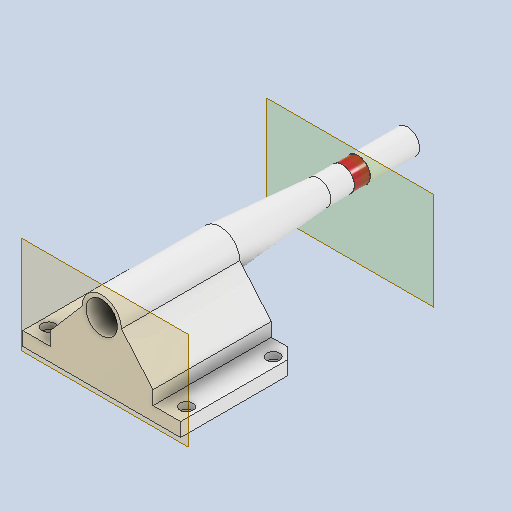
# Autodesk Inventor part: Guide
Saved by Autodesk Inventor 2024 (Build 280153000, 153)
## iProperties
Created: 2021-10-05
Part Number: Guide
Material: PBT-Kunststoff
Document SubType Name: Modeling
Designer: espen
Density: 1.31 g/cm^3
Appearance: Glatt - Weiß
Mass: 141.322 g
Surface Area: 254.19 cm^2
Volume: 107.879 cm^3
ToolGuidance_Base_Thickness: 7,000 mm
Guidacne_fixHoleDist: 70,000 mm
Author: espen
Autodesk Inventor part; units mm, degrees
ref_plane "YZ Plane" through (0, 0, 0) normal (1, 0, 0) x (0, 1, 0)
ref_plane "XZ Plane" through (0, 0, 0) normal (0, 1, 0) x (-1, 0, 0)
ref_plane "XY Plane" through (0, 0, 0) normal (0, 0, 1) x (1, 0, 0)
sketch "Sketch1" plane through (0, 0, 0) normal (0, 0, 1) x (1, 0, 0)
  arc A0 (10, 32.7) -> (-10, 32.7) centre (0, 32.7) ccw
  line L0 (-10, 32.7) -> (-26, 14)
  line L1 (-26, 14) -> (-26, 7)
  line L2 (-26, 7) -> (-40, 7)
  line L3 (-40, 7) -> (-40, 0)
  line L4 (-40, 0) -> (0, 0)
  line L5 (0, 32.7) -> (0, 0) construction
  line L6 (10, 32.7) -> (26, 14)
  line L7 (26, 14) -> (26, 7)
  line L8 (26, 7) -> (40, 7)
  line L9 (40, 7) -> (40, 0)
  line L10 (40, 0) -> (0, 0)
  line L11 (-10, 32.7) -> (10, 32.7) construction
  dimension "d4" = 10
  dimension "d5" = 80
  dimension "ToolGuidance_Base_Thickness" = 7
  dimension "d7" = 7
  dimension "d8" = 32.7
  dimension "d9" = 14
  dimension "d11" = 0
  constraints: 24 end point, 4 symmetric about line, 3 perpendicular, 2 point on circle, 2 vertical, 1 centre point, 1 coincident, 1 horizontal, 1 midpoint, 1 point on line
  measures "d4" radius of A0
  measures "d5" diameter of L3 L5
  measures "ToolGuidance_Base_Thickness" distance between parallel lines of L8 L10
  measures "d7" distance from line of L6.end L8
  measures "d8" distance from line of L10 A0.centre
  measures "d9" distance between parallel lines of L7 L9
  measures "d11" distance from line of L4.end L5
extrude "Extrusion1" add sketch "Sketch1" against normal blind 60
sketch "Sketch2" plane through (0, 0, 0) normal (0, 0, 1) x (1, 0, 0)
  arc A0 (10, 32.7) -> (-10, 32.7) centre (0, 32.7) ccw projected
  circle A1 centre (0, 32.7) radius 8
  point P0 (0, 0)
  dimension "d16" = 16
  constraints: 1 centre point, 1 coincident
  measures "d16" diameter of A1
extrude "Extrusion2" cut sketch "Sketch2" against normal blind 20
sketch "Sketch3" plane through (0, 0, -60) normal (0, 0, -1) x (-1, 0, 0)
  circle A0 centre (0, 32.7) radius 8 projected
  circle A1 centre (0, 32.7) radius 4.25
  point P0 (0, 0)
  dimension "d19" = 8.5
  constraints: 1 centre point, 1 coincident
  measures "d19" diameter of A1
extrude "Extrusion3" cut sketch "Sketch3" against normal blind 60 contours A1
sketch "Sketch4" plane through (-40, 7, 0) normal (0, 1, 0) x (1, 0, 0)
  circle A0 centre (5, 52) radius 2.25 construction
  line L0 (0, 60) -> (14, 60) construction
  line L1 (0, 0) -> (0, 60) construction
  circle A1 centre (5, 8) radius 2.25 construction
  line L2 (96, 0) -> (-16, 0) construction
  line L3 (40, 60) -> (40, 0) construction
  circle A2 centre (75, 52) radius 2.25 construction
  circle A3 centre (75, 8) radius 2.25 construction
  line L4 (80, 0) -> (80, 60) construction
  line L5 (66, 60) -> (80, 60) construction
  line L6 (75, 52) -> (75, 8) construction
  line L7 (5, 52) -> (5, 8) construction
  line L8 (0, 0) -> (0, 60) construction
  point P0 (73, 60)
  point P1 (7, 60)
  dimension "d25" = 4.5
  dimension "d26" = 8
  dimension "d28" = 4.5
  dimension "d29" = 8
  dimension "d54" = 44
  dimension "Guidacne_fixHoleDist" = 70
  constraints: 6 end point, 4 centre point, 4 coincident, 2 midpoint, 2 symmetric about line, 1 parallel, 1 point on line, 1 vertical, 2 other
  measures "d25" diameter of A0
  measures "d26" distance from line of A0.centre L0
  measures "d28" diameter of A1
  measures "d29" distance from line of A1.centre L2
  measures "d54" distance of A0.centre A1.centre
  measures "Guidacne_fixHoleDist" distance between parallel lines of L6 L7
hole "Bohrung1" at (35, 7, -52) at (35, 7, -8) at (-35, 7, -8) at (-35, 7, -52) direction (0, -1, 0) diameter 3.4 end through all counterbore diameter 6.5 counterbore depth 3.4 clearance for "Inbusschraube DIN EN ISO 4762" size "M3" standard "DIN"
sketch "Sketch5" plane through (0, 0, 0) normal (1, 0, 0) x (0, 1, 0)
  line L0 (32.7, 0) -> (32.7, -60) projected
  line L1 (32.7, 0) -> (32.7, -180.9299)
  line L2 (32.7, -60) -> (42.7, -60) projected
  line L3 (42.7, -60) -> (38.95, -110)
  line L4 (38.95, -110) -> (38.95, -155)
  line L5 (36.95, -60) -> (36.95, -20) projected
  line L6 (36.95, -60) -> (36.95, -155)
  line L7 (36.95, -155) -> (38.95, -155)
  line L8 (42.7, 0) -> (32.7, 0) projected
  point P0 (0, 0)
  dimension "d34" = 2
  dimension "d35" = 155
  dimension "d36" = 110
  constraints: 10 end point, 2 perpendicular, 2 point on line, 1 collinear, 1 parallel
  measures "d34" distance between parallel lines of L6 L4
  measures "d35" distance from line of L4.end L8
  measures "d36" distance from line of L3.end L8
revolve "Revolution1" add sketch "Sketch5" angle 360 about axis through (0, 32.7, 0) along (0, 0, -1)
sketch "Sketch6" plane through (0, 0, 0) normal (1, 0, 0) x (0, 1, 0)
  line L0 (32.7, 0) -> (32.7, -60) projected
  line L1 (32.7, -41.8536) -> (32.7, 16.9969)
  line L2 (24.7, -20) -> (40.7, -20) projected
  line L3 (40.7, -20) -> (36.95, -33.9952)
  line L4 (36.95, -155) -> (36.95, -20) projected
  line L5 (28.45, -20) -> (36.95, -20) projected
  line L6 (36.95, -33.9952) -> (36.95, -20)
  line L7 (36.95, -20) -> (40.7, -20)
  line L8 (36.95, -33.9952) -> (36.95, -20)
  line L9 (40.7, -20) -> (36.95, -20)
  point P0 (0, 0)
  dimension "d38" = 15
  constraints: 12 end point, 2 collinear, 2 perpendicular, 2 point on line, 1 vertical
  measures "d38" angle of L4 L3
revolve "Revolution2" cut sketch "Sketch6" angle 360 about axis through (0, 32.7, -41.8536) along (0, 0, 1)
sketch "Sketch7" plane through (0, 0, 0) normal (1, 0, 0) x (0, 1, 0)
  line L0 (26.45, -110) -> (38.95, -110) projected
  line L1 (32.7, -110) -> (32.7, -160.0229)
  line L2 (38.95, -110) -> (38.95, -155) projected
  line L3 (38.95, -122) -> (38.85, -122)
  line L4 (38.85, -122) -> (38.85, -130)
  line L5 (38.85, -130) -> (38.95, -130)
  line L6 (38.95, -130) -> (38.95, -122)
  line L7 (42.7, 0) -> (32.7, 0) projected
  point P0 (0, 0)
  dimension "d40" = 0.1
  dimension "d41" = 122
  dimension "d42" = 8
  constraints: 10 end point, 2 parallel, 1 horizontal, 1 midpoint, 1 perpendicular, 1 point on line, 1 vertical
  measures "d40" distance of L3.start L3.end
  measures "d41" distance from line of L7 L3.start
  measures "d42" distance of L4.end L3.end
revolve "Revolution3" cut sketch "Sketch7" angle 360 about axis through (0, 32.7, -110) along (0, 0, -1)
ref_plane "Arbeitsebene1" through (0, 32.7, -126) normal (0, 0, -1) x (-1, 0, 0)
ref_plane "Arbeitsebene2" through (26, 7, 0) normal (0, 0, 1) x (1, 0, 0)
chamfer "Fase2" distance 6 angle 45 2 edges at (-40, 3.5, -60) (40, 3.5, -60)
equation "\"d5\" = GuidanceTrac_Width"
equation "\"d25\" = d28"
equation "\"GuidanceTrac_Width\" = 80"
body "Solid1"
